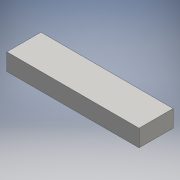
# Autodesk Inventor part: 240626_chair7
Saved by Autodesk Inventor 2016 (Build 200138000, 138)
## iProperties
Created: 2024-06-26
Part Number: 240626_chair7
Material: 일반
Document SubType Name: Modeling
Designer: pc
Density: 1 g/cm^3
Appearance: 기본값
Author: pc
Autodesk Inventor part; units mm, degrees
ref_plane "YZ Plane" through (0, 0, 0) normal (1, 0, 0) x (0, 1, 0)
ref_plane "XZ Plane" through (0, 0, 0) normal (0, 1, 0) x (-1, 0, 0)
ref_plane "XY Plane" through (0, 0, 0) normal (0, 0, 1) x (1, 0, 0)
sketch "스케치1" plane through (0, 0, 0) normal (0, 0, 1) x (1, 0, 0)
  line L0 (19.4055, -5) -> (-19.4055, -5)
  line L1 (-19.4055, -5) -> (-19.4055, 5)
  line L2 (-19.4055, 5) -> (19.4055, 5)
  line L3 (19.4055, 5) -> (19.4055, -5)
  line L4 (19.4055, -5) -> (-19.4055, 5) construction
  line L5 (-19.4055, -5) -> (19.4055, 5) construction
  point P0 (0, 0)
  dimension "d0" = 38.811
  dimension "d1" = 10
  constraints: 12 end point, 2 midpoint, 2 parallel, 1 horizontal, 1 perpendicular
  measures "d0" distance of L1.end L2.end
  measures "d1" distance of L0.end L1.end
extrude "돌출1" add sketch "스케치1" along normal blind 5
